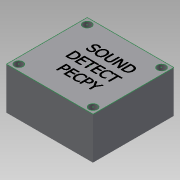
# Autodesk Inventor part: SoundDetectBaru
Saved by Autodesk Inventor 2015 SP1 (Build 190203100, 203)
## iProperties
Created: 2015-02-01
Part Number: SoundDetectBaru
Material: Generic
Document SubType Name: Modeling
Designer: Rafi Kurnia Putra
Density: 1 g/cm^3
Appearance: Default
Mass: 12.9234 g
Surface Area: 40.795 cm^2
Volume: 12.9234 cm^3
Author: Rafi Kurnia Putra
Autodesk Inventor part; units mm, degrees
ref_plane "YZ Plane" through (0, 0, 0) normal (1, 0, 0) x (0, 1, 0)
ref_plane "XZ Plane" through (0, 0, 0) normal (0, 1, 0) x (-1, 0, 0)
ref_plane "XY Plane" through (0, 0, 0) normal (0, 0, 1) x (1, 0, 0)
sketch "Sketch1" plane through (0, 0, 0) normal (0, 1, 0) x (-1, 0, 0)
  line L0 (15.4432, 14.405) -> (-15.4432, 14.405)
  line L1 (-15.4432, 14.405) -> (-15.4432, -14.405)
  line L2 (-15.4432, -14.405) -> (15.4432, -14.405)
  line L3 (15.4432, -14.405) -> (15.4432, 14.405)
  circle A0 centre (13.2432, -12.205) radius 1.5
  circle A1 centre (13.2432, 12.205) radius 1.5
  circle A2 centre (-13.2428, -12.205) radius 1.5
  circle A3 centre (-13.2428, 12.205) radius 1.5
  point P0 (0, 0)
  dimension "d0" = 30.8864
  dimension "d1" = 28.81
  dimension "d2" = 3
  dimension "d6" = 2.2
  dimension "d7" = 2.2
  dimension "d16" = 24.41
  dimension "d19" = 26.486
  constraints: 8 end point, 4 centre point, 3 horizontal, 2 parallel, 2 vertical, 1 perpendicular, 6 other
  measures "d0" distance of L2.end L1.end
  measures "d1" distance of L1.end L0.end
  measures "d2" diameter of A0
  measures "d6" distance from line of L3 A0.centre
  measures "d7" distance from line of L2 A0.centre
  measures "d16" distance of A0.centre A1.centre
  measures "d19" distance of A0.centre A2.centre
extrude "Extrusion1" add sketch "Sketch1" along normal blind 15
sketch "Sketch2" plane through (0, 0, 0) normal (0, -1, 0) x (1, 0, 0)
  circle A0 centre (13.2428, 12.205) radius 1.5 projected
  circle A1 centre (13.2428, -12.205) radius 1.5 projected
  circle A2 centre (-13.2432, 12.205) radius 1.5 projected
  circle A3 centre (-13.2432, -12.205) radius 1.5 projected
  line L0 (-15.4432, 14.405) -> (15.4432, 14.405) projected
  line L1 (-15.4432, -14.405) -> (-15.4432, 14.405) projected
  line L2 (15.4432, -14.405) -> (-15.4432, -14.405) projected
  line L3 (15.4432, 14.405) -> (15.4432, -14.405) projected
  circle A4 centre (13.2428, -12.205) radius 1.5 projected
  line L4 (13.2428, -12.205) -> (-13.2432, 12.205)
  circle A5 centre (-13.2432, -12.205) radius 1.5 projected
  line L5 (13.2428, 12.205) -> (-13.2432, -12.205)
  point P0 (0, 0)
  constraints: 4 end point
sketch "Sketch3" plane through (0, 15, 0) normal (0, 1, 0) x (1, 0, 0)
  circle A0 centre (13.2428, -12.205) radius 1.5 projected
  circle A1 centre (13.2428, 12.205) radius 1.5 projected
  circle A2 centre (-13.2432, -12.205) radius 1.5 projected
  circle A3 centre (-13.2432, 12.205) radius 1.5 projected
  line L0 (-15.4432, -14.405) -> (15.4432, -14.405) projected
  line L1 (15.4432, -14.405) -> (15.4432, 14.405) projected
  line L2 (15.4432, 14.405) -> (-15.4432, 14.405) projected
  line L3 (-15.4432, 14.405) -> (-15.4432, -14.405) projected
  line L4 (23.1035, -2.0134) -> (-26.5318, -2.0134) construction
  line L5 (-26.5318, -2.0134) -> (-26.5318, 1.4328) construction
  line L6 (-26.5318, 1.4328) -> (23.1035, 1.4328) construction
  line L7 (23.1035, 1.4328) -> (23.1035, -2.0134) construction
  point P0 (0, 0)
  constraints: 2 other
body "Solid1"
